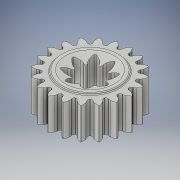
# Autodesk Inventor part: gear sleeve
Saved by Autodesk Inventor 2017 (Build 210142000, 142)
## iProperties
Created: 2020-09-28
Part Number: gear sleeve
Material: Generic
Document SubType Name: Modeling
Designer: Brandt
Density: 1 g/cm^3
Appearance: Default
Author: Brandt
Autodesk Inventor part; units mm, degrees
ref_plane "YZ Plane" through (0, 0, 0) normal (1, 0, 0) x (0, 1, 0)
ref_plane "XZ Plane" through (0, 0, 0) normal (0, 1, 0) x (-1, 0, 0)
ref_plane "XY Plane" through (0, 0, 0) normal (0, 0, 1) x (1, 0, 0)
sketch "Sketch10" plane through (0, 0, 0) normal (0, 1, 0) x (-1, 0, 0)
  circle A0 centre (0, 0) radius 5.9626 construction
  circle A1 centre (0, 0) radius 5.2737
  dimension "d40" = 11.9253
  dimension "d43" = 0.689
  constraints: 2 centre point, 2 coincident
  measures "d40" diameter of A0
  measures "d43" radial gap between concentric circles of A0 A1
extrude "Extrusion9" add sketch "Sketch10" along normal blind 5.461
sketch "Sketch11" plane through (0, 5.461, 0) normal (0, 1, 0) x (1, 0, 0)
  circle A0 centre (0, 0) radius 5.2737
  line L0 (0, 0) -> (0, 20.1574) construction
  arc A1 (0.0381, 6.5436) -> (-0.0381, 6.5436) centre (0, 0) ccw
  arc A2 (-0.0381, 6.5436) -> (-0.4496, 5.9535) centre (1.2694, 5.1933) ccw
  arc A3 (0.4496, 5.9535) -> (0.0381, 6.5436) centre (-1.2694, 5.1933) ccw
  line L1 (0.4496, 5.9535) -> (-0.4496, 5.9535) construction
  arc A4 (-0.4496, 5.9535) -> (-0.5382, 5.6131) centre (0.5493, 5.5117) ccw
  line L2 (0, 0) -> (-0.365, 3.7729) construction
  line L3 (0, 0) -> (0.3566, 3.6861) construction
  line L4 (0.5079, 5.2492) -> (0.5381, 5.5614)
  line L5 (-0.5079, 5.2492) -> (-0.5381, 5.5614)
  arc A5 (-0.5382, 5.6131) -> (-0.5381, 5.5614) centre (-0.2661, 5.5878) ccw
  arc A6 (0.5381, 5.5614) -> (0.5382, 5.6131) centre (0.2661, 5.5878) ccw
  line L6 (0.698, 5.2273) -> (-0.698, 5.2273)
  line L7 (0.2661, 5.5878) -> (-0.2661, 5.5878) construction
  circle A7 centre (0, 0) radius 5.2737 projected
  arc A8 (0.5382, 5.6131) -> (0.4496, 5.9535) centre (-0.5493, 5.5117) ccw
  point P0 (-0.2562, 2.6483)
  point P1 (0.1816, 1.8766)
  dimension "d71" = 1.396
  dimension "d72" = 0.0762
  dimension "d73" = 0.0381
  dimension "d74" = 6.5437
  dimension "d75" = 0.698
  dimension "d76" = 1.8796
  dimension "d77" = 1.8796
  dimension "d78" = 0.8992
  dimension "d79" = 1.0922
  dimension "d81" = 0.2733
  dimension "d82" = 0.4496
  dimension "d83" = 0.3657
  dimension "d84" = 0.5321
  dimension "d85" = 0.2661
  dimension "d86" = 0.5901
  dimension "d87" = 11.053
  dimension "d95" = 1.0922
  constraints: 18 point on circle, 16 end point, 8 centre point, 7 tangent, 6 point on line, 4 coincident, 2 horizontal, 1 concentric, 1 vertical
  measures "d71" distance of L6.end L6.start
  measures "d72" distance of A1.end A3.end
  measures "d73" distance from line of L0 A1.end
  measures "d74" radius of A1
  measures "d75" horizontal distance of L0.start L6.start
  measures "d76" radius of A2
  measures "d77" radius of A3
  measures "d78" distance of L1.start L1.end
  measures "d79" radius of A4
  measures "d81" radius of A5
  measures "d82" horizontal distance of point (0, 0) L1.start
  measures "d83" distance from line of L1 L7.end
  measures "d84" distance of L7.start L7.end
  measures "d85" distance from line of L0 L7.start
  measures "d86" distance from line of L1 A1.end
  measures "d87" angle of L3 L2
  measures "d95" radius of A8
extrude "Extrusion10" add sketch "Sketch11" against normal up to surface (5.461 mm away) contours A0 L5 A5 A4 A2 A1 A3 A8 A6 L4
fillet "Fillet5" radius 0.3175 2 edges at (-0.5079, 2.7305, -5.2492) (0.5079, 2.7305, -5.2492)
pattern_circular "Circular Pattern4" count 20 over 360 about axis through (0, 0, 0) along (0, 1, 0) of "Extrusion10", "Fillet5"
sketch "Sketch12" plane through (0, 0, 0) normal (0, -1, 0) x (-1, 0, 0)
  arc A0 (-1.0187, 1.6285) -> (-1.0516, 1.6075) centre (0, 0) ccw construction
  arc A1 (-1.4637, 1.6634) -> (-1.0516, 1.6075) centre (-1.2254, 1.8732) ccw construction
  line L0 (-1.4637, 1.6634) -> (-1.4758, 1.6771) construction
  arc A2 (-1.4758, 1.6771) -> (-1.5461, 1.7343) centre (-1.6809, 1.4966) ccw construction
  arc A3 (-1.5461, 1.7343) -> (-1.876, 1.8563) centre (-2.085, 0.7843) ccw construction
  arc A4 (-1.876, 1.8563) -> (-2.5953, 1.8563) centre (-2.2357, 0.0114) ccw construction
  arc A5 (-2.5953, 1.8563) -> (-2.6389, 1.7938) centre (0, 0) ccw construction
  arc A6 (-2.6389, 1.7938) -> (-2.3903, 1.1188) centre (-0.7834, 2.0939) ccw construction
  arc A7 (-2.3903, 1.1188) -> (-2.1618, 0.8514) centre (-1.4566, 1.6854) ccw construction
  arc A8 (-2.1618, 0.8514) -> (-2.0838, 0.8052) centre (-1.9853, 1.0601) ccw construction
  line L1 (-2.0838, 0.8052) -> (-2.0668, 0.7986) construction
  arc A9 (-1.8719, 0.4312) -> (-2.0668, 0.7986) centre (-2.1813, 0.5024) ccw construction
  arc A10 (-1.8719, 0.4312) -> (-1.8802, 0.3931) centre (0, 0) ccw construction
  arc A11 (-2.2112, 0.1412) -> (-1.8802, 0.3931) centre (-2.191, 0.4581) ccw construction
  line L2 (-2.2112, 0.1412) -> (-2.2294, 0.1424) construction
  arc A12 (-2.2294, 0.1424) -> (-2.3196, 0.1331) centre (-2.2468, -0.1304) ccw construction
  arc A13 (-2.3196, 0.1331) -> (-2.6391, -0.0139) centre (-2.0289, -0.9197) ccw construction
  arc A14 (-2.6391, -0.0139) -> (-3.1478, -0.5226) centre (-1.5889, -1.5728) ccw construction
  arc A15 (-3.1478, -0.5226) -> (-3.1344, -0.5976) centre (0, 0) ccw construction
  arc A16 (-3.1344, -0.5976) -> (-2.4813, -0.8991) centre (-2.0346, 0.9266) ccw construction
  arc A17 (-2.4813, -0.8991) -> (-2.1306, -0.9266) centre (-2.2217, 0.1618) ccw construction
  arc A18 (-2.1306, -0.9266) -> (-2.0428, -0.9042) centre (-2.1534, -0.6542) ccw construction
  line L3 (-2.0428, -0.9042) -> (-2.0262, -0.8968) construction
  arc A19 (-1.6285, -1.0187) -> (-2.0262, -0.8968) centre (-1.8977, -1.1871) ccw construction
  arc A20 (-1.6285, -1.0187) -> (-1.6075, -1.0516) centre (0, 0) ccw construction
  arc A21 (-1.6634, -1.4637) -> (-1.6075, -1.0516) centre (-1.8732, -1.2254) ccw construction
  line L4 (-1.6634, -1.4637) -> (-1.6771, -1.4758) construction
  arc A22 (-1.6771, -1.4758) -> (-1.7343, -1.5461) centre (-1.4966, -1.6809) ccw construction
  arc A23 (-1.7343, -1.5461) -> (-1.8563, -1.876) centre (-0.7843, -2.085) ccw construction
  arc A24 (-1.8563, -1.876) -> (-1.8563, -2.5953) centre (-0.0114, -2.2357) ccw construction
  arc A25 (-1.8563, -2.5953) -> (-1.7938, -2.6389) centre (0, 0) ccw construction
  arc A26 (-1.7938, -2.6389) -> (-1.1188, -2.3903) centre (-2.0939, -0.7834) ccw construction
  arc A27 (-1.1188, -2.3903) -> (-0.8514, -2.1618) centre (-1.6854, -1.4566) ccw construction
  arc A28 (-0.8514, -2.1618) -> (-0.8052, -2.0838) centre (-1.0601, -1.9853) ccw construction
  line L5 (-0.8052, -2.0838) -> (-0.7986, -2.0668) construction
  arc A29 (-0.4312, -1.8719) -> (-0.7986, -2.0668) centre (-0.5024, -2.1813) ccw construction
  arc A30 (-0.4312, -1.8719) -> (-0.3931, -1.8802) centre (0, 0) ccw construction
  arc A31 (-0.1412, -2.2112) -> (-0.3931, -1.8802) centre (-0.4581, -2.191) ccw construction
  line L6 (-0.1412, -2.2112) -> (-0.1424, -2.2294) construction
  arc A32 (-0.1424, -2.2294) -> (-0.1331, -2.3196) centre (0.1304, -2.2468) ccw construction
  arc A33 (-0.1331, -2.3196) -> (0.0139, -2.6391) centre (0.9197, -2.0289) ccw construction
  arc A34 (0.0139, -2.6391) -> (0.5226, -3.1478) centre (1.5728, -1.5889) ccw construction
  arc A35 (0.5226, -3.1478) -> (0.5976, -3.1344) centre (0, 0) ccw construction
  arc A36 (0.5976, -3.1344) -> (0.8991, -2.4813) centre (-0.9266, -2.0346) ccw construction
  arc A37 (0.8991, -2.4813) -> (0.9266, -2.1306) centre (-0.1618, -2.2217) ccw construction
  arc A38 (0.9266, -2.1306) -> (0.9042, -2.0428) centre (0.6542, -2.1534) ccw construction
  line L7 (0.9042, -2.0428) -> (0.8968, -2.0262) construction
  arc A39 (1.0187, -1.6285) -> (0.8968, -2.0262) centre (1.1871, -1.8977) ccw construction
  arc A40 (1.0187, -1.6285) -> (1.0516, -1.6075) centre (0, 0) ccw construction
  arc A41 (1.4637, -1.6634) -> (1.0516, -1.6075) centre (1.2254, -1.8732) ccw construction
  line L8 (1.4637, -1.6634) -> (1.4758, -1.6771) construction
  arc A42 (1.4758, -1.6771) -> (1.5461, -1.7343) centre (1.6809, -1.4966) ccw construction
  arc A43 (1.5461, -1.7343) -> (1.876, -1.8563) centre (2.085, -0.7843) ccw construction
  arc A44 (1.876, -1.8563) -> (2.5953, -1.8563) centre (2.2357, -0.0114) ccw construction
  arc A45 (2.5953, -1.8563) -> (2.6389, -1.7938) centre (0, 0) ccw construction
  arc A46 (2.6389, -1.7938) -> (2.3903, -1.1188) centre (0.7834, -2.0939) ccw construction
  arc A47 (2.3903, -1.1188) -> (2.1618, -0.8514) centre (1.4566, -1.6854) ccw construction
  arc A48 (2.1618, -0.8514) -> (2.0838, -0.8052) centre (1.9853, -1.0601) ccw construction
  line L9 (2.0838, -0.8052) -> (2.0668, -0.7986) construction
  arc A49 (1.8719, -0.4312) -> (2.0668, -0.7986) centre (2.1813, -0.5024) ccw construction
  arc A50 (1.8719, -0.4312) -> (1.8802, -0.3931) centre (0, 0) ccw construction
  arc A51 (2.2112, -0.1412) -> (1.8802, -0.3931) centre (2.191, -0.4581) ccw construction
  line L10 (2.2112, -0.1412) -> (2.2294, -0.1424) construction
  arc A52 (2.2294, -0.1424) -> (2.3196, -0.1331) centre (2.2468, 0.1304) ccw construction
  arc A53 (2.3196, -0.1331) -> (2.6391, 0.0139) centre (2.0289, 0.9197) ccw construction
  arc A54 (2.6391, 0.0139) -> (3.1478, 0.5226) centre (1.5889, 1.5728) ccw construction
  arc A55 (3.1478, 0.5226) -> (3.1344, 0.5976) centre (0, 0) ccw construction
  arc A56 (3.1344, 0.5976) -> (2.4813, 0.8991) centre (2.0346, -0.9266) ccw construction
  arc A57 (2.4813, 0.8991) -> (2.1306, 0.9266) centre (2.2217, -0.1618) ccw construction
  arc A58 (2.1306, 0.9266) -> (2.0428, 0.9042) centre (2.1534, 0.6542) ccw construction
  line L11 (2.0428, 0.9042) -> (2.0262, 0.8968) construction
  arc A59 (1.6285, 1.0187) -> (2.0262, 0.8968) centre (1.8977, 1.1871) ccw construction
  arc A60 (1.6285, 1.0187) -> (1.6075, 1.0516) centre (0, 0) ccw construction
  arc A61 (1.6634, 1.4637) -> (1.6075, 1.0516) centre (1.8732, 1.2254) ccw construction
  line L12 (1.6634, 1.4637) -> (1.6771, 1.4758) construction
  arc A62 (1.6771, 1.4758) -> (1.7343, 1.5461) centre (1.4966, 1.6809) ccw construction
  arc A63 (1.7343, 1.5461) -> (1.8563, 1.876) centre (0.7843, 2.085) ccw construction
  arc A64 (1.8563, 1.876) -> (1.8563, 2.5953) centre (0.0114, 2.2357) ccw construction
  arc A65 (1.8563, 2.5953) -> (1.7938, 2.6389) centre (0, 0) ccw construction
  arc A66 (1.7938, 2.6389) -> (1.1188, 2.3903) centre (2.0939, 0.7834) ccw construction
  arc A67 (1.1188, 2.3903) -> (0.8514, 2.1618) centre (1.6854, 1.4566) ccw construction
  arc A68 (0.8514, 2.1618) -> (0.8052, 2.0838) centre (1.0601, 1.9853) ccw construction
  line L13 (0.8052, 2.0838) -> (0.7986, 2.0668) construction
  arc A69 (0.4312, 1.8719) -> (0.7986, 2.0668) centre (0.5024, 2.1813) ccw construction
  arc A70 (0.4312, 1.8719) -> (0.3931, 1.8802) centre (0, 0) ccw construction
  arc A71 (0.1412, 2.2112) -> (0.3931, 1.8802) centre (0.4581, 2.191) ccw construction
  line L14 (0.1412, 2.2112) -> (0.1424, 2.2294) construction
  arc A72 (0.1424, 2.2294) -> (0.1331, 2.3196) centre (-0.1304, 2.2468) ccw construction
  arc A73 (0.1331, 2.3196) -> (-0.0139, 2.6391) centre (-0.9197, 2.0289) ccw construction
  arc A74 (-0.0139, 2.6391) -> (-0.5226, 3.1478) centre (-1.5728, 1.5889) ccw construction
  arc A75 (-0.5226, 3.1478) -> (-0.5976, 3.1344) centre (0, 0) ccw construction
  arc A76 (-0.5976, 3.1344) -> (-0.8991, 2.4813) centre (0.9266, 2.0346) ccw construction
  arc A77 (-0.8991, 2.4813) -> (-0.9266, 2.1306) centre (0.1618, 2.2217) ccw construction
  arc A78 (-0.9266, 2.1306) -> (-0.9042, 2.0428) centre (-0.6542, 2.1534) ccw construction
  line L15 (-0.9042, 2.0428) -> (-0.8968, 2.0262) construction
  arc A79 (-1.0187, 1.6285) -> (-0.8968, 2.0262) centre (-1.1871, 1.8977) ccw construction
  circle A80 centre (0, 0) radius 8.0242 construction
  arc A81 (-2.4121, -4.6897) -> (-2.3763, -4.708) centre (0, 0) ccw projected
  line L16 (-2.1126, 0.6801) -> (-2.1296, 0.6867)
  arc A82 (-2.2438, 0.7544) -> (-2.1296, 0.6867) centre (-1.9853, 1.0601) ccw
  arc A83 (-2.4989, 1.0529) -> (-2.2438, 0.7544) centre (-1.4566, 1.6854) ccw
  arc A84 (-2.7718, 1.8236) -> (-2.4989, 1.0529) centre (-0.7834, 2.0939) ccw
  arc A85 (-2.6693, 1.9706) -> (-2.7718, 1.8236) centre (0, 0) ccw
  arc A86 (-1.8517, 1.981) -> (-2.6693, 1.9706) centre (-2.2357, 0.0114) ccw
  arc A87 (-1.4834, 1.8448) -> (-1.8517, 1.981) centre (-2.085, 0.7843) ccw
  arc A88 (-1.3804, 1.761) -> (-1.4834, 1.8448) centre (-1.6809, 1.4966) ccw
  line L17 (-1.3804, 1.761) -> (-1.3684, 1.7473)
  arc A89 (-1.3684, 1.7473) -> (-1.1211, 1.7138) centre (-1.2254, 1.8732) ccw
  arc A90 (-1.0861, 1.7361) -> (-1.1211, 1.7138) centre (0, 0) ccw
  arc A91 (-1.0861, 1.7361) -> (-1.0129, 1.9748) centre (-1.1871, 1.8977) ccw
  line L18 (-1.0129, 1.9748) -> (-1.0203, 1.9914)
  arc A92 (-1.0532, 2.12) -> (-1.0203, 1.9914) centre (-0.6542, 2.1534) ccw
  arc A93 (-1.0225, 2.5115) -> (-1.0532, 2.12) centre (0.1618, 2.2217) ccw
  arc A94 (-0.6704, 3.2494) -> (-1.0225, 2.5115) centre (0.9266, 2.0346) ccw
  arc A95 (-0.494, 3.2809) -> (-0.6704, 3.2494) centre (0, 0) ccw
  arc A96 (0.0914, 2.7101) -> (-0.494, 3.2809) centre (-1.5728, 1.5889) ccw
  arc A97 (0.2555, 2.3534) -> (0.0914, 2.7101) centre (-0.9197, 2.0289) ccw
  arc A98 (0.2691, 2.2213) -> (0.2555, 2.3534) centre (-0.1304, 2.2468) ccw
  line L19 (0.2691, 2.2213) -> (0.268, 2.2031)
  arc A99 (0.268, 2.2031) -> (0.4191, 2.0045) centre (0.4581, 2.191) ccw
  arc A100 (0.4597, 1.9956) -> (0.4191, 2.0045) centre (0, 0) ccw
  arc A101 (0.4597, 1.9956) -> (0.6801, 2.1126) centre (0.5024, 2.1813) ccw
  line L20 (0.6801, 2.1126) -> (0.6867, 2.1296)
  arc A102 (0.7544, 2.2438) -> (0.6867, 2.1296) centre (1.0601, 1.9853) ccw
  arc A103 (1.0529, 2.4989) -> (0.7544, 2.2438) centre (1.6854, 1.4566) ccw
  arc A104 (1.8236, 2.7718) -> (1.0529, 2.4989) centre (2.0939, 0.7834) ccw
  arc A105 (1.9706, 2.6693) -> (1.8236, 2.7718) centre (0, 0) ccw
  arc A106 (1.981, 1.8517) -> (1.9706, 2.6693) centre (0.0114, 2.2357) ccw
  arc A107 (1.8448, 1.4834) -> (1.981, 1.8517) centre (0.7843, 2.085) ccw
  arc A108 (1.761, 1.3804) -> (1.8448, 1.4834) centre (1.4966, 1.6809) ccw
  line L21 (1.761, 1.3804) -> (1.7473, 1.3684)
  arc A109 (1.7473, 1.3684) -> (1.7138, 1.1211) centre (1.8732, 1.2254) ccw
  arc A110 (1.7361, 1.0861) -> (1.7138, 1.1211) centre (0, 0) ccw
  arc A111 (1.7361, 1.0861) -> (1.9748, 1.0129) centre (1.8977, 1.1871) ccw
  line L22 (1.9748, 1.0129) -> (1.9914, 1.0203)
  arc A112 (2.12, 1.0532) -> (1.9914, 1.0203) centre (2.1534, 0.6542) ccw
  arc A113 (2.5115, 1.0225) -> (2.12, 1.0532) centre (2.2217, -0.1618) ccw
  arc A114 (3.2494, 0.6704) -> (2.5115, 1.0225) centre (2.0346, -0.9266) ccw
  arc A115 (3.2809, 0.494) -> (3.2494, 0.6704) centre (0, 0) ccw
  arc A116 (2.7101, -0.0914) -> (3.2809, 0.494) centre (1.5889, 1.5728) ccw
  arc A117 (2.3534, -0.2555) -> (2.7101, -0.0914) centre (2.0289, 0.9197) ccw
  arc A118 (2.2213, -0.2691) -> (2.3534, -0.2555) centre (2.2468, 0.1304) ccw
  line L23 (2.2213, -0.2691) -> (2.2031, -0.268)
  arc A119 (2.2031, -0.268) -> (2.0045, -0.4191) centre (2.191, -0.4581) ccw
  arc A120 (1.9956, -0.4597) -> (2.0045, -0.4191) centre (0, 0) ccw
  arc A121 (1.9956, -0.4597) -> (2.1126, -0.6801) centre (2.1813, -0.5024) ccw
  line L24 (2.1126, -0.6801) -> (2.1296, -0.6867)
  arc A122 (2.2438, -0.7544) -> (2.1296, -0.6867) centre (1.9853, -1.0601) ccw
  arc A123 (2.4989, -1.0529) -> (2.2438, -0.7544) centre (1.4566, -1.6854) ccw
  arc A124 (2.7718, -1.8236) -> (2.4989, -1.0529) centre (0.7834, -2.0939) ccw
  arc A125 (2.6693, -1.9706) -> (2.7718, -1.8236) centre (0, 0) ccw
  arc A126 (1.8517, -1.981) -> (2.6693, -1.9706) centre (2.2357, -0.0114) ccw
  arc A127 (1.4834, -1.8448) -> (1.8517, -1.981) centre (2.085, -0.7843) ccw
  arc A128 (1.3804, -1.761) -> (1.4834, -1.8448) centre (1.6809, -1.4966) ccw
  line L25 (1.3804, -1.761) -> (1.3684, -1.7473)
  arc A129 (1.3684, -1.7473) -> (1.1211, -1.7138) centre (1.2254, -1.8732) ccw
  arc A130 (1.0861, -1.7361) -> (1.1211, -1.7138) centre (0, 0) ccw
  arc A131 (1.0861, -1.7361) -> (1.0129, -1.9748) centre (1.1871, -1.8977) ccw
  line L26 (1.0129, -1.9748) -> (1.0203, -1.9914)
  arc A132 (1.0532, -2.12) -> (1.0203, -1.9914) centre (0.6542, -2.1534) ccw
  arc A133 (1.0225, -2.5115) -> (1.0532, -2.12) centre (-0.1618, -2.2217) ccw
  arc A134 (0.6704, -3.2494) -> (1.0225, -2.5115) centre (-0.9266, -2.0346) ccw
  arc A135 (0.494, -3.2809) -> (0.6704, -3.2494) centre (0, 0) ccw
  arc A136 (-0.0914, -2.7101) -> (0.494, -3.2809) centre (1.5728, -1.5889) ccw
  arc A137 (-0.2555, -2.3534) -> (-0.0914, -2.7101) centre (0.9197, -2.0289) ccw
  arc A138 (-0.2691, -2.2213) -> (-0.2555, -2.3534) centre (0.1304, -2.2468) ccw
  line L27 (-0.2691, -2.2213) -> (-0.268, -2.2031)
  arc A139 (-0.268, -2.2031) -> (-0.4191, -2.0045) centre (-0.4581, -2.191) ccw
  arc A140 (-0.4597, -1.9956) -> (-0.4191, -2.0045) centre (0, 0) ccw
  arc A141 (-0.4597, -1.9956) -> (-0.6801, -2.1126) centre (-0.5024, -2.1813) ccw
  line L28 (-0.6801, -2.1126) -> (-0.6867, -2.1296)
  arc A142 (-0.7544, -2.2438) -> (-0.6867, -2.1296) centre (-1.0601, -1.9853) ccw
  arc A143 (-1.0529, -2.4989) -> (-0.7544, -2.2438) centre (-1.6854, -1.4566) ccw
  arc A144 (-1.8236, -2.7718) -> (-1.0529, -2.4989) centre (-2.0939, -0.7834) ccw
  arc A145 (-1.9706, -2.6693) -> (-1.8236, -2.7718) centre (0, 0) ccw
  arc A146 (-1.981, -1.8517) -> (-1.9706, -2.6693) centre (-0.0114, -2.2357) ccw
  arc A147 (-1.8448, -1.4834) -> (-1.981, -1.8517) centre (-0.7843, -2.085) ccw
  arc A148 (-1.761, -1.3804) -> (-1.8448, -1.4834) centre (-1.4966, -1.6809) ccw
  line L29 (-1.761, -1.3804) -> (-1.7473, -1.3684)
  arc A149 (-1.7473, -1.3684) -> (-1.7138, -1.1211) centre (-1.8732, -1.2254) ccw
  arc A150 (-1.7361, -1.0861) -> (-1.7138, -1.1211) centre (0, 0) ccw
  arc A151 (-1.7361, -1.0861) -> (-1.9748, -1.0129) centre (-1.8977, -1.1871) ccw
  line L30 (-1.9748, -1.0129) -> (-1.9914, -1.0203)
  arc A152 (-2.12, -1.0532) -> (-1.9914, -1.0203) centre (-2.1534, -0.6542) ccw
  arc A153 (-2.5115, -1.0225) -> (-2.12, -1.0532) centre (-2.2217, 0.1618) ccw
  arc A154 (-3.2494, -0.6704) -> (-2.5115, -1.0225) centre (-2.0346, 0.9266) ccw
  arc A155 (-3.2809, -0.494) -> (-3.2494, -0.6704) centre (0, 0) ccw
  arc A156 (-2.7101, 0.0914) -> (-3.2809, -0.494) centre (-1.5889, -1.5728) ccw
  arc A157 (-2.3534, 0.2555) -> (-2.7101, 0.0914) centre (-2.0289, -0.9197) ccw
  arc A158 (-2.2213, 0.2691) -> (-2.3534, 0.2555) centre (-2.2468, -0.1304) ccw
  line L31 (-2.2213, 0.2691) -> (-2.2031, 0.268)
  arc A159 (-2.2031, 0.268) -> (-2.0045, 0.4191) centre (-2.191, 0.4581) ccw
  arc A160 (-1.9956, 0.4597) -> (-2.0045, 0.4191) centre (0, 0) ccw
  arc A161 (-1.9956, 0.4597) -> (-2.1126, 0.6801) centre (-2.1813, 0.5024) ccw
  point P0 (0, 0)
  dimension "d71" = 1.396
  dimension "d72" = 0.0762
  dimension "d73" = 0.0381
  dimension "d74" = 6.5437
  dimension "d75" = 0.698
  dimension "d76" = 1.8796
  dimension "d77" = 1.8796
  dimension "d78" = 0.8992
  dimension "d79" = 1.0922
  dimension "d81" = 0.2733
  dimension "d82" = 0.4496
  dimension "d83" = 0.3657
  dimension "d84" = 0.5321
  dimension "d85" = 0.2661
  dimension "d86" = 0.5901
  dimension "d87" = 11.053
  dimension "d95" = 1.0922
  dimension "d100" = 0.127
  constraints: 320 point on circle, 161 centre point, 64 end point, 1 concentric, 95 other
  measures "d100" radial gap between concentric circles of A9 A161
extrude "Extrusion11" cut sketch "Sketch12" against normal through all
sketch "Sketch13" plane through (0, 0, 0) normal (1, 0, 0) x (0, 1, 0)
  line L0 (5.461, 0) -> (3.8828, 0)
  line L1 (3.8828, 0) -> (5.461, -3.81)
  line L2 (5.461, -3.81) -> (5.461, 0)
  line L3 (-1.0922, 0) -> (6.5532, 0) projected
  line L4 (5.461, -4.1791) -> (5.461, -3.7432) projected
  point P0 (0, 0)
  point P1 (5.461, 1.9956)
  dimension "d106" = 22.5
  dimension "d108" = 3.81
  dimension "d109" = 0
  constraints: 6 end point, 1 horizontal, 1 point on line, 1 vertical
  measures "d106" angle of L1 L2
  measures "d108" distance from line of L3 L1.end
  measures "d109" distance from line of L1.end L4
revolve "Revolution1" cut sketch "Sketch13" angle 360 about axis through (0, -10, 0) along (0, 1, 0)
sketch "Sketch14" plane through (0, 5.461, 0) normal (0, 1, 0) x (1, 0, 0)
  circle A0 centre (0, 0) radius 4.445
  circle A1 centre (0, 0) radius 12.7
  dimension "d110" = 8.89
  dimension "d111" = 25.4
  constraints: 2 centre point, 2 coincident
  measures "d110" diameter of A0
  measures "d111" diameter of A1
extrude "Extrusion12" cut sketch "Sketch14" against normal blind 0.254
sketch "Sketch15" plane through (0, 0, 0) normal (0, -1, 0) x (1, 0, 0)
  circle A0 centre (0, 0) radius 4.445
  circle A1 centre (0, 0) radius 12.7
  dimension "d114" = 8.89
  dimension "d115" = 25.4
  constraints: 2 centre point, 2 coincident
  measures "d114" diameter of A0
  measures "d115" diameter of A1
extrude "Extrusion13" cut sketch "Sketch15" against normal blind 0.254
fillet "Fillet6" radius 0.127 4 edges at (-4.445, 0.254, 0) (-4.445, 0, 0) (-4.445, 5.207, 0) (-4.445, 5.461, 0)
equation "\"Bottom_Ratio\" = 0.333333"
equation "\"Pitch\" = 45.454545"
equation "\"Offset\" = 0.7493"
equation "\"d61\" = 0.7493"
equation "\"d62\" = 45.454545"
equation "\"Top_Ratio\" = 0.25"
equation "\"d89\" = 0.7493"
equation "\"d90\" = 45.454545"
equation "\"SunPitchDiam\" = 11.9253"
body "Solid1"
